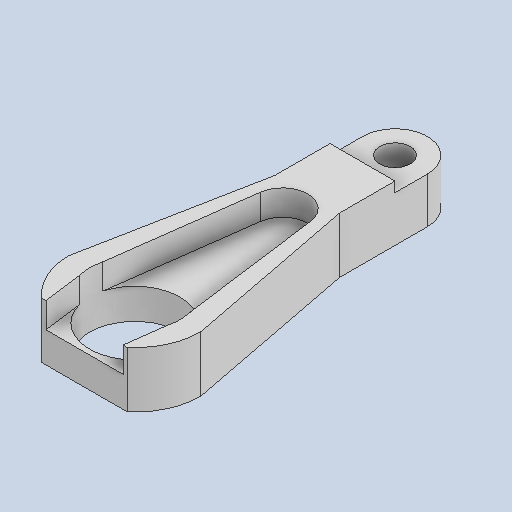
# Autodesk Inventor part: Servo_Exzenter_Smart_Neu_2
Saved by Autodesk Inventor 2023 (Build 270158000, 158)
## iProperties
Created: 2022-04-12
Part Number: Servo_Exzenter_Smart_Neu_2
Material: Generisch
Document SubType Name: Modeling
Designer: trist
Density: 1 g/cm^3
Appearance: Vorgabe
Author: trist
Autodesk Inventor part; units mm, degrees
ref_plane "YZ Plane" through (0, 0, 0) normal (1, 0, 0) x (0, 1, 0)
ref_plane "XZ Plane" through (0, 0, 0) normal (0, 1, 0) x (-1, 0, 0)
ref_plane "XY Plane" through (0, 0, 0) normal (0, 0, 1) x (1, 0, 0)
sketch "Skizze1" plane through (0, 0, 0) normal (0, 1, 0) x (-1, 0, 0)
  circle A0 centre (0, 0) radius 4.45
  arc A1 (6.5, 0) -> (-6.5, 0) centre (0, 0) ccw
  line L0 (0, 0) -> (0, -17)
  line L1 (4, -14) -> (23.7753, -14) construction
  line L2 (0, 0) -> (0, -19.75)
  line L3 (0, 0) -> (0, -26.15)
  line L4 (0, 0) -> (0, -29.15)
  arc A2 (-3.2, -29.15) -> (3.2, -29.15) centre (0, -29.15) ccw
  line L5 (-3.2, -29.15) -> (-3.2, -24.95)
  line L6 (3.2, -29.15) -> (3.2, -26.15)
  line L7 (3.2, -26.15) -> (3.2, -17)
  line L8 (-3.2, -24.95) -> (-3.2, -23.5465)
  line L9 (-3.2, -23.5465) -> (-3.2, -17)
  line L10 (-3.2, -17) -> (-6.5, 0)
  line L11 (6.5, 0) -> (3.2, -17)
  line L12 (0, -29.15) -> (0, -25.65)
  arc A3 (-3.2, -25.65) -> (3.2, -25.65) centre (0, -25.65) ccw
  point P0 (3.2, -25.65)
  dimension "d0" = 8.9
  dimension "d1" = 13
  dimension "d2" = 17
  dimension "d27" = 6.4
  dimension "d35" = 3.5
  constraints: 26 end point, 7 point on line, 6 point on circle, 4 centre point, 4 coincident, 2 tangent, 2 vertical, 1 horizontal, 1 parallel, 1 symmetric about line
  measures "d0" diameter of A0
  measures "d1" diameter of A1
  measures "d2" distance of L0.start L0.end
  measures "d27" diameter of A2
  measures "d35" distance of L12.start L12.end
extrude "Extrusion1" add sketch "Skizze1" along normal blind 3 contours A3 L5 L8 L9 L10 A1 L11 L7
sketch "Skizze2" plane through (0, 3, 0) normal (0, 1, 0) x (1, 0, 0)
  arc A0 (-6.5, 0) -> (6.5, 0) centre (0, 0) ccw projected
  line L0 (-3.2, 17) -> (-3.2, 19.75)
  line L1 (3.2, 17) -> (3.2, 19.75)
  line L2 (3.2, 26.15) -> (3.2, 19.75)
  line L3 (-3.2, 26.15) -> (-3.2, 19.75)
  arc A1 (3.2, 29.15) -> (-3.2, 29.15) centre (0, 29.15) ccw
  line L4 (3.2, 26.15) -> (3.2, 29.15)
  line L5 (-3.2, 26.15) -> (-3.2, 29.15)
  arc A2 (-6.5, 0) -> (6.5, 0) centre (0, 0) ccw
  line L6 (-3.2, 29.15) -> (-3.2, 17) projected
  line L7 (-6.5, 0) -> (-3.2, 17)
  line L8 (6.5, 0) -> (3.2, 17) projected
  line L9 (6.5, 0) -> (3.2, 17)
  circle A3 centre (0, 0) radius 4.45
  circle A4 centre (0, 0) radius 4.45 projected
  line L10 (0, -4.45) -> (0, 14.55)
  arc A5 (2.482, 14.8497) -> (-2.482, 14.8497) centre (0, 14.55) ccw
  line L11 (-4.45, 0) -> (-2.4744, 14.9071)
  line L12 (4.45, 0) -> (2.4744, 14.9071)
  line L13 (-4.45, 0) -> (4.45, 0)
  line L14 (-4.45, 0) -> (-3.746, -5.312)
  line L15 (4.45, 0) -> (3.746, -5.312)
  arc A6 (3.2, 29.15) -> (-3.2, 29.15) centre (0, 29.15) ccw projected
  arc A7 (3.2, 25.65) -> (-3.2, 25.65) centre (0, 25.65) ccw projected
  arc A8 (3.2, 25.65) -> (-3.2, 25.65) centre (0, 25.65) ccw
  point P0 (-4.0763, 3.9842)
  point P1 (-5.7, 0)
  point P2 (0, 19.75)
  point P3 (-3.2, 26.15)
  point P4 (-2.4744, -14.9071)
  point P5 (2.4744, -14.9071)
  point P6 (-4.2964, -1.1592)
  point P7 (-4.2964, 1.1592)
  point P8 (4.2964, 1.1592)
  point P9 (4.2964, -1.1592)
  point P10 (3.2, 17)
  point P11 (-3.2, 26.65)
  point P12 (3.2, 26.65)
  dimension "d30" = 19
  dimension "d31" = 5
  constraints: 28 end point, 13 point on circle, 8 point on line, 5 centre point, 4 coincident, 4 symmetric about line, 3 vertical, 1 collinear, 1 concentric, 1 horizontal
  measures "d30" distance of L10.start L10.end
  measures "d31" diameter of A5
extrude "Extrusion2" add sketch "Skizze2" along normal blind 2.5 contours L7 L0 L3 A7 L2 L1 L8 A0 L15 A3 L12 A5 L11 L14
sketch "Skizze5" plane through (0, 0, 0) normal (0, -1, 0) x (1, 0, 0)
  line L0 (0, 0) -> (0, -29.15)
  circle A0 centre (0, -29.15) radius 1.5
  arc A1 (-3.2, -25.65) -> (3.2, -25.65) centre (0, -25.65) ccw projected
  line L1 (0, -29.15) -> (0, -25.65)
  circle A2 centre (0, -25.65) radius 1.5
  point P0 (-3.2, -26.65)
  dimension "d20" = 29.15
  dimension "d21" = 3
  dimension "d40" = 3.5
  dimension "d41" = 3
  constraints: 4 end point, 2 centre point, 2 coincident, 1 collinear, 1 vertical
  measures "d20" distance of L0.start L0.end
  measures "d21" diameter of A0
  measures "d40" distance of L1.start L1.end
  measures "d41" diameter of A2
extrude "Extrusion5" cut sketch "Skizze5" against normal blind 6 contours A2 L0 | L0 A2
sketch "Skizze6" plane through (0, 5.5, 0) normal (0, 1, 0) x (1, 0, 0)
  arc A0 (3.2, 29.15) -> (-3.2, 29.15) centre (0, 29.15) ccw
  line L0 (-3.2, 29.15) -> (-3.2, 14) projected
  line L1 (-3.2, 29.15) -> (-3.2, 25.9472)
  arc A1 (3.2, 29.15) -> (-3.2, 29.15) centre (0, 29.15) ccw projected
  line L2 (3.2, 29.15) -> (3.2, 25.9472)
  line L3 (-3.2, 25.9472) -> (-3.2, 23.4472)
  line L4 (-3.2, 25.65) -> (-3.2, 17) projected
  line L5 (3.2, 17) -> (3.2, 25.65) projected
  arc A2 (3.2, 25.65) -> (-3.2, 25.65) centre (0, 25.65) ccw projected
  arc A3 (3.2, 26.65) -> (-3.2, 26.65) centre (0, 26.65) ccw
  line L6 (3.2, 17) -> (3.2, 25.65) projected
  line L7 (3.2, 26.65) -> (3.2, 23.4472)
  line L8 (-3.2, 23.4472) -> (-3.2, 22.4472)
  line L9 (-3.2, 25.65) -> (-3.2, 17) projected
  line L10 (-3.2, 22.4472) -> (3.2, 22.4472)
  line L11 (3.2, 23.4472) -> (3.2, 22.4472)
  point P0 (0, 0)
  dimension "d38" = 2.5
  dimension "d43" = 1
  constraints: 14 end point, 6 point on line, 4 point on circle, 3 tangent, 2 centre point, 2 collinear, 2 perpendicular, 1 coincident, 1 vertical alignment
  measures "d38" distance of L1.end L3.end
  measures "d43" distance of L3.end L8.end
extrude "Extrusion6" cut sketch "Skizze6" against normal blind 1
sketch "Skizze7" plane through (0, 0, 0) normal (0, -1, 0) x (1, 0, 0)
  circle A0 centre (0, 0) radius 4.45 projected
  line L0 (-6.6957, 4.45) -> (-6.6957, 6.6948)
  line L1 (-6.6957, 6.6948) -> (6.8805, 6.6948)
  line L2 (6.8805, 6.6948) -> (6.8805, 4.45)
  line L3 (6.8805, 4.45) -> (6.8805, 4.95)
  line L4 (6.8805, 4.95) -> (-6.6957, 4.95)
  dimension "d34" = 0.5
  constraints: 10 end point, 2 point on line, 1 parallel, 1 perpendicular
  measures "d34" distance of L2.end L3.end
extrude "Extrusion7" cut sketch "Skizze7" against normal blind 20 contours L0 L1 L2 L4
